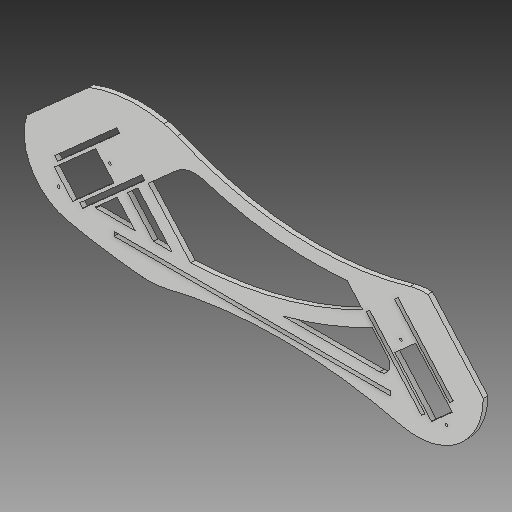
# Autodesk Inventor part: Cuerpo - Lateral
Saved by Autodesk Inventor 2019 (Build 230136000, 136)
## iProperties
Created: 2020-02-14
Part Number: Cuerpo - Lateral
Material: Genérico
Document SubType Name: Modeling
Designer: Mafer1
Density: 1 g/cm^3
Appearance: Valor por defecto
Mass: 61.885 g
Surface Area: 460.37 cm^2
Volume: 61.885 cm^3
base_servo: 20.000 mm
altura_servo: 40.000 mm
agujero_servo: 2.000 mm
distancia_agujero_servo: 4.750 mm
soporte: 60.000 mm
largo_base: 200.000 mm
Author: Mafer1
Autodesk Inventor part; units mm, degrees
ref_plane "YZ Plane" through (0, 0, 0) normal (1, 0, 0) x (0, 1, 0)
ref_plane "XZ Plane" through (0, 0, 0) normal (0, 1, 0) x (-1, 0, 0)
ref_plane "XY Plane" through (0, 0, 0) normal (0, 0, 1) x (1, 0, 0)
sketch "Boceto2" plane through (0, 0, 0) normal (0, 0, 1) x (1, 0, 0)
  circle A0 centre (0, 0) radius 40
  circle A1 centre (-200, 0) radius 52.5
  circle A2 centre (-250, -5) radius 40
  arc A3 (-258.4353, -44.1005) -> (-204.7198, -52.2874) centre (-164.804, 389.9147) ccw
  arc A4 (-188.9974, 51.3341) -> (-279.8859, 21.5863) centre (-208.9069, -41.5562) ccw
  arc A5 (-179.4312, 48.3029) -> (-11.2392, 38.3885) centre (-81.4844, 278.3169) ccw
  arc A6 (-46.5935, -31) -> (31.225, 25) centre (-6.245, -5) ccw
  arc A7 (-18.0162, -51.5343) -> (-187.4585, -50.98) centre (-103.8482, -390.8466) ccw
  dimension "d42" = 80
  dimension "d43" = 200
  dimension "d44" = 105
  dimension "d45" = 80
  dimension "d46" = 50
  dimension "d47" = 5
  dimension "d48" = 444
  dimension "d49" = 95
  dimension "d50" = 250
  dimension "d51" = 350
  dimension "d52" = 5
  dimension "d53" = 48
  dimension "d54" = 31
  constraints: 19 point on circle, 9 tangent, 8 centre point, 1 coincident, 1 horizontal alignment
  measures "d42" diameter of A0
  measures "d43" distance of point (0, 0) A1.centre
  measures "d44" diameter of A1
  measures "d45" diameter of A2
  measures "d46" horizontal distance of A1.centre A2.centre
  measures "d47" vertical distance of A2.centre A1.centre
  measures "d48" radius of A3
  measures "d49" radius of A4
  measures "d50" radius of A5
  measures "d51" radius of A7
  measures "d52" vertical distance of point (0, 0) A6.centre
  measures "d53" radius of A6
  measures "d54" vertical distance of point (0, 0) A6.start
extrude "Extrusión1" add sketch "Boceto2" along normal blind 3.3
sketch "Boceto3" plane through (0, 0, 3.3) normal (0, 0, 1) x (1, 0, 0)
  arc A0 (-179.4312, 48.3029) -> (-11.2392, 38.3885) centre (-81.4844, 278.3169) ccw projected
  arc A1 (31.225, 25) -> (-11.2392, 38.3885) centre (0, 0) ccw projected
  arc A2 (-179.4312, 48.3029) -> (-11.2392, 38.3885) centre (-81.4844, 278.3169) ccw projected
  arc A3 (-179.4312, 48.3029) -> (-188.9974, 51.3341) centre (-200, 0) ccw projected
  arc A4 (-188.9974, 51.3341) -> (-279.8859, 21.5863) centre (-208.9069, -41.5562) ccw projected
  arc A5 (-279.8859, 21.5863) -> (-258.4353, -44.1005) centre (-250, -5) ccw projected
  arc A6 (-258.4353, -44.1005) -> (-204.7198, -52.2874) centre (-164.804, 389.9147) ccw projected
  arc A7 (-204.7198, -52.2874) -> (-187.4585, -50.98) centre (-200, 0) ccw projected
  arc A8 (-18.0162, -51.5343) -> (-187.4585, -50.98) centre (-103.8482, -390.8466) ccw projected
  arc A9 (-18.0162, -51.5343) -> (31.225, 25) centre (-6.245, -5) ccw projected
  arc A10 (-18.0162, -51.5343) -> (31.225, 25) centre (-6.245, -5) ccw projected
  arc A11 (31.225, 25) -> (-11.2392, 38.3885) centre (0, 0) ccw projected
  line L0 (1.755, 39.9615) -> (41.755, -5.0385)
  arc A12 (-279.8859, 21.5863) -> (-258.4353, -44.1005) centre (-250, -5) ccw projected
  line L1 (-288.1379, 7.0623) -> (-243.1379, 47.0623)
  arc A13 (-188.9974, 51.3341) -> (-279.8859, 21.5863) centre (-208.9069, -41.5562) ccw projected
  line L2 (-7.2418, 4.9269) -> (19.3327, -24.9694)
  line L3 (19.3327, -24.9694) -> (4.3845, -38.2567)
  line L4 (4.3845, -38.2567) -> (-22.19, -8.3603)
  line L5 (-22.19, -8.3603) -> (-7.2418, 4.9269)
  line L6 (-268.207, -15.36) -> (-254.9197, -30.3082)
  line L7 (-254.9197, -30.3082) -> (-225.0234, -3.7336)
  line L8 (-225.0234, -3.7336) -> (-238.3106, 11.2146)
  line L9 (-268.207, -15.36) -> (-238.3106, 11.2146)
  line L10 (-265.7987, -10.5434) -> (-220.9541, 29.3185)
  line L11 (-223.1465, 31.7849) -> (-267.9911, -8.0769)
  line L12 (-249.854, -28.4812) -> (-205.0094, 11.3807)
  line L13 (-205.0094, 11.3807) -> (-202.817, 8.9142)
  line L14 (-202.817, 8.9142) -> (-247.6616, -30.9476)
  line L15 (-247.6616, -30.9476) -> (-249.854, -28.4812)
  circle A14 centre (-230.359, 4.9031) radius 1
  circle A15 centre (-262.8713, -23.9967) radius 1
  line L16 (-22.3561, 24.9409) -> (17.5057, -19.9037)
  line L17 (17.5057, -19.9037) -> (19.9722, -17.7113)
  line L18 (19.9722, -17.7113) -> (-19.8897, 27.1333)
  line L19 (-19.8897, 27.1333) -> (-22.3561, 24.9409)
  line L20 (-40.2939, 8.9962) -> (-0.4321, -35.8484)
  line L21 (-0.4321, -35.8484) -> (-2.8986, -38.0408)
  line L22 (-2.8986, -38.0408) -> (-42.7604, 6.8038)
  line L23 (-42.7604, 6.8038) -> (-40.2939, 8.9962)
  circle A16 centre (-15.8786, -0.4087) radius 1
  circle A17 centre (13.0213, -32.921) radius 1
  arc A18 (-18.0162, -51.5343) -> (-187.4585, -50.98) centre (-103.8482, -390.8466) ccw projected
  line L24 (-220.9541, 29.3185) -> (-223.1465, 31.7849)
  line L25 (-267.9911, -8.0769) -> (-265.7987, -10.5434)
  line L26 (-253.2588, -2.0727) -> (-239.9715, -17.0209) construction
  line L27 (-8.9028, -23.3085) -> (6.0454, -10.0212) construction
  line L28 (-225, -34) -> (-25, -34)
  line L29 (-25, -34) -> (-25, -37)
  line L30 (-25, -37) -> (-225, -37)
  line L31 (-225, -37) -> (-225, -34)
  dimension "d59" = 40
  dimension "d60" = 45
  dimension "d61" = 40
  dimension "d62" = 45
  dimension "d65" = 40
  dimension "d66" = 20
  dimension "d68" = 30
  dimension "d69" = 0
  dimension "d70" = 40
  dimension "d71" = 20
  dimension "d73" = 30
  dimension "d74" = 0
  dimension "d75" = 2
  dimension "d76" = 2
  dimension "d77" = 3.3
  dimension "d78" = 3.3
  dimension "d80" = 60
  dimension "d84" = 2
  dimension "d85" = 2
  dimension "d86" = 1.75
  dimension "d87" = 10
  dimension "d88" = 1.75
  dimension "d89" = 10
  dimension "d90" = 2
  dimension "d91" = 2
  dimension "d94" = 3.3
  dimension "d95" = 3.3
  dimension "d96" = 60
  dimension "d97" = 60
  dimension "d98" = 2
  dimension "d99" = 10
  dimension "d100" = 10
  dimension "d101" = 1.75
  dimension "d102" = 1.75
  dimension "d103" = 60
  dimension "d105" = 15
  dimension "d106" = 15
  dimension "d107" = 15
  dimension "d108" = 15
  dimension "d109" = 3
  dimension "d110" = 34
  dimension "d111" = 200
  dimension "d112" = 25
  constraints: 64 end point, 19 perpendicular, 4 centre point, 4 midpoint, 4 point on circle, 3 parallel, 1 equal radius, 1 horizontal
  measures "d59" horizontal distance of L0.start L0.end
  measures "d60" vertical distance of L0.start L0.end
  measures "d61" vertical distance of L1.start L1.end
  measures "d62" horizontal distance of L1.start L1.end
  measures "d65" distance of L3.end L4.end
  measures "d66" distance from line of L4 L2.start
  measures "d68" distance between parallel lines of L0 L2
  measures "d69" distance from line of L0.end L3
  measures "d70" distance between parallel lines of L6 L8
  measures "d71" distance between parallel lines of L9 L7
  measures "d73" distance between parallel lines of L9 L1
  measures "d74" distance from line of L6 L1.start
  measures "d75" distance between parallel lines of L9 L10
  measures "d76" distance between parallel lines of L12 L7
  measures "d77" distance between parallel lines of L10 L11
  measures "d78" distance between parallel lines of L12 L14
  measures "d80" distance between parallel lines of L13 L15
  measures "d84" diameter of A14
  measures "d85" diameter of A15
  measures "d86" distance from line of L8 A14.centre
  measures "d87" distance from line of L7 A14.centre
  measures "d88" distance from line of L6 A15.centre
  measures "d89" distance from line of L9 A15.centre
  measures "d90" distance between parallel lines of L2 L16
  measures "d91" distance between parallel lines of L20 L4
  measures "d94" distance between parallel lines of L16 L18
  measures "d95" distance between parallel lines of L22 L20
  measures "d96" distance between parallel lines of L17 L19
  measures "d97" distance between parallel lines of L21 L23
  measures "d98" diameter of A16
  measures "d99" distance from line of L2 A16.centre
  measures "d100" distance from line of A17.centre L2
  measures "d101" distance from line of L5 A16.centre
  measures "d102" distance from line of L3 A17.centre
  measures "d103" distance between parallel lines of L25 L24
  measures "d105" distance between parallel lines of L25 L26
  measures "d106" distance between parallel lines of L27 L17
  measures "d107" distance between parallel lines of L21 L27
  measures "d108" distance between parallel lines of L15 L26
  measures "d109" distance between parallel lines of L30 L28
  measures "d110" distance from line of A1.centre L28
  measures "d111" distance between parallel lines of L29 L31
  measures "d112" horizontal distance of L28.end A1.centre
extrude "Extrusión2" cut sketch "Boceto3" against normal blind 3.3 contours A1 A9 L0 | L1 A5 A4 | L2 L3 L4 L5 | L9 L8 L7 L6 | L25 L11 L24 L10 | L12 L13 L14 L15 | A14 | A15 | L19 L18 L17 L16 | L20 L21 L22 L23 | A16 | A17 | L28 L29 L30 L31
sketch "Sketch4" plane through (0, 0, 3.3) normal (0, 0, 1) x (1, 0, 0)
  arc A0 (-179.4312, 48.3029) -> (-11.2392, 38.3885) centre (-81.4844, 278.3169) ccw projected
  line L0 (-225, -34) -> (-25, -34) projected
  arc A1 (-179.4312, 48.3029) -> (-188.9974, 51.3341) centre (-200, 0) ccw projected
  arc A2 (-188.9974, 51.3341) -> (-243.1379, 47.0623) centre (-208.9069, -41.5562) ccw projected
  line L1 (-209.9139, -26) -> (-238.1379, -26)
  line L2 (41.755, -5.0385) -> (1.755, 39.9615) projected
  arc A3 (1.755, 39.9615) -> (-11.2392, 38.3885) centre (0, 0) ccw projected
  arc A4 (-179.4312, 48.3029) -> (-11.2392, 38.3885) centre (-81.4844, 278.3169) ccw projected
  arc A5 (-179.4312, 48.3029) -> (-188.9974, 51.3341) centre (-200, 0) ccw projected
  arc A6 (-188.9974, 51.3341) -> (-243.1379, 47.0623) centre (-208.9069, -41.5562) ccw projected
  line L3 (-243.1379, 47.0623) -> (-288.1379, 7.0623) projected
  arc A7 (-288.1379, 7.0623) -> (-258.4353, -44.1005) centre (-250, -5) ccw projected
  arc A8 (-258.4353, -44.1005) -> (-204.7198, -52.2874) centre (-164.804, 389.9147) ccw projected
  arc A9 (-204.7198, -52.2874) -> (-187.4585, -50.98) centre (-200, 0) ccw projected
  arc A10 (-18.0162, -51.5343) -> (-187.4585, -50.98) centre (-103.8482, -390.8466) ccw projected
  arc A11 (-18.0162, -51.5343) -> (41.755, -5.0385) centre (-6.245, -5) ccw projected
  line L4 (-225.0234, -3.7336) -> (-254.9197, -30.3082) projected
  line L5 (-254.9197, -30.3082) -> (-268.207, -15.36) projected
  line L6 (-268.207, -15.36) -> (-238.3106, 11.2146) projected
  line L7 (-238.3106, 11.2146) -> (-225.0234, -3.7336) projected
  line L8 (-247.6616, -30.9476) -> (-249.854, -28.4812) projected
  line L9 (-249.854, -28.4812) -> (-205.0094, 11.3807) projected
  line L10 (-205.0094, 11.3807) -> (-202.817, 8.9142) projected
  line L11 (-202.817, 8.9142) -> (-247.6616, -30.9476) projected
  line L12 (19.9722, -17.7113) -> (17.5057, -19.9037) projected
  line L13 (17.5057, -19.9037) -> (-22.3561, 24.9409) projected
  line L14 (-22.3561, 24.9409) -> (-19.8897, 27.1333) projected
  line L15 (-19.8897, 27.1333) -> (19.9722, -17.7113) projected
  circle A12 centre (13.0213, -32.921) radius 1 projected
  circle A13 centre (-262.8713, -23.9967) radius 1 projected
  circle A14 centre (-230.359, 4.9031) radius 1 projected
  circle A15 centre (-15.8786, -0.4087) radius 1 projected
  line L16 (-42.7604, 6.8038) -> (-40.2939, 8.9962) projected
  line L17 (-40.2939, 8.9962) -> (-0.4321, -35.8484) projected
  line L18 (-0.4321, -35.8484) -> (-2.8986, -38.0408) projected
  line L19 (-2.8986, -38.0408) -> (-42.7604, 6.8038) projected
  line L20 (-223.1465, 31.7849) -> (-220.9541, 29.3185) projected
  line L21 (-220.9541, 29.3185) -> (-265.7987, -10.5434) projected
  line L22 (-265.7987, -10.5434) -> (-267.9911, -8.0769) projected
  line L23 (-267.9911, -8.0769) -> (-223.1465, 31.7849) projected
  line L24 (-22.19, -8.3603) -> (-7.2418, 4.9269) projected
  line L25 (-7.2418, 4.9269) -> (19.3327, -24.9694) projected
  line L26 (19.3327, -24.9694) -> (4.3845, -38.2567) projected
  line L27 (4.3845, -38.2567) -> (-22.19, -8.3603) projected
  line L28 (-225, -37) -> (-225, -34) projected
  line L29 (-225, -34) -> (-25, -34) projected
  line L30 (-25, -34) -> (-25, -37) projected
  line L31 (-25, -37) -> (-225, -37) projected
  line L32 (-202.817, 8.9142) -> (-247.6616, -30.9476) projected
  arc A16 (-238.3772, -25.3707) -> (-238.1379, -26) centre (-238.1379, -25.6399) ccw
  line L33 (-238.3772, -25.3707) -> (-222.7894, -11.515)
  line L34 (-222.7894, -11.515) -> (-209.9139, -26)
  line L35 (-196.5343, -26) -> (-215.3153, -4.8713)
  line L36 (-215.3153, -4.8713) -> (-207.8412, 1.7723)
  line L37 (-207.8412, 1.7723) -> (-183.1548, -26)
  line L38 (-183.1548, -26) -> (-196.5343, -26)
  line L39 (-200.3672, 8.4159) -> (-169.7752, -26)
  line L40 (-200.3672, 8.4159) -> (-179.974, 26.5432)
  arc A17 (-160.6008, 30.6466) -> (-179.974, 26.5432) centre (-166.6867, 11.595) ccw
  arc A18 (-160.6008, 30.6466) -> (-56.7209, 19.4989) centre (-81.4844, 278.3169) ccw
  line L41 (-56.7209, 19.4989) -> (-45.4609, 6.8314)
  arc A19 (-103.245, -26) -> (-38.6081, -0.8779) centre (-182.2347, 272.9473) ccw
  line L42 (-267.9911, -8.0769) -> (-223.1465, 31.7849) projected
  arc A20 (-18.0162, -51.5343) -> (41.755, -5.0385) centre (-6.245, -5) ccw projected
  line L43 (-103.245, -26) -> (-33.245, -26)
  arc A21 (-33.245, -26) -> (-27.5501, -13.3183) centre (-33.245, -18.3804) ccw
  line L44 (-38.6081, -0.8779) -> (-27.5501, -13.3183)
  line L45 (-2.8986, -38.0408) -> (-42.7604, 6.8038) projected
  line L46 (-42.7604, 6.8038) -> (-40.2939, 8.9962) projected
  arc A22 (-169.7752, -26) -> (-45.4609, 6.8314) centre (-182.2347, 272.9473) ccw
  line L47 (-223.1465, 31.7849) -> (-220.9541, 29.3185) projected
  dimension "d113" = 10
  dimension "d114" = 10
  dimension "d115" = 10
  dimension "d117" = 10
  dimension "d119" = 50
  dimension "d121" = 10
  dimension "d126" = 10
  dimension "d129" = 10
  dimension "d130" = 75
  dimension "d131" = 70
  dimension "d132" = 20
  dimension "d136" = 10
  dimension "d139" = 10
  constraints: 24 end point, 12 point on circle, 7 point on line, 6 centre point, 6 tangent, 4 parallel, 2 collinear, 2 concentric, 2 horizontal, 2 perpendicular, 2 other
  measures "d114" distance between parallel lines of L35 L34
  measures "d115" distance between parallel lines of L39 L37
  measures "d119" horizontal distance of A16.centre L3.end
  measures "d121" distance between parallel lines of L37 L35
  measures "d126" radial gap between concentric circles of A18 A0
  measures "d130" horizontal distance of L2.start A21.centre
  measures "d131" distance of L43.start L43.end
  measures "d132" radius of A17
  measures "d136" radial gap between concentric circles of A22 A19
extrude "Extrusión5" cut sketch "Sketch4" against normal blind 10 contours L1 A16 L33 L34 | L35 L36 L37 L38 | L40 A17 A18 L41 A22 L39 | A19 L44 A21 L43
equation "\"d45\" = d42"
equation "\"d65\" = altura_servo"
equation "\"d66\" = base_servo"
equation "\"d70\" = d65"
equation "\"d71\" = d66"
equation "\"d78\" = d77"
equation "\"d84\" = agujero_servo"
equation "\"d85\" = d84"
equation "\"d87\" = 0.5 * d71"
equation "\"d88\" = d86"
equation "\"d89\" = 0.5 * d71"
equation "\"d91\" = d90"
equation "\"d95\" = d94"
equation "\"d97\" = d96"
equation "\"d98\" = agujero_servo"
equation "\"d99\" = 0.5 * d66"
equation "\"d100\" = d99"
equation "\"d102\" = d101"
equation "\"soporte\" = 60"
equation "\"largo_base\" = 200"
equation "\"altura_servo\" = 40"
equation "\"base_servo\" = 20"
equation "\"agujero_servo\" = 2"
